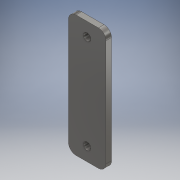
# Autodesk Inventor part: SIDE BEARING GUIDE
Saved by Autodesk Inventor 2018 (Build 220112000, 112)
## iProperties
Created: 2018-10-05
Part Number: SIDE BEARING GUIDE
Material: Acero
Document SubType Name: Modeling
Designer: Toshiba
Density: 7.85 g/cm^3
Appearance: Semipulido
Author: Toshiba
Autodesk Inventor part; units mm, degrees
ref_plane "YZ Plane" through (0, 0, 0) normal (1, 0, 0) x (0, 1, 0)
ref_plane "XZ Plane" through (0, 0, 0) normal (0, 1, 0) x (-1, 0, 0)
ref_plane "XY Plane" through (0, 0, 0) normal (0, 0, 1) x (1, 0, 0)
sketch "Boceto3" plane through (0, 0, 0) normal (0, 0, 1) x (1, 0, 0)
  line L0 (20, -3) -> (20, 3)
  line L1 (20, 3) -> (-20, 3)
  line L2 (-20, 3) -> (-20, -3)
  line L3 (-20, -3) -> (20, -3)
  line L4 (20, -3) -> (-20, 3) construction
  line L5 (20, 3) -> (-20, -3) construction
  point P0 (0, 0)
  dimension "d15" = 6
  dimension "d16" = 40
  constraints: 12 end point, 2 midpoint, 2 parallel, 1 perpendicular, 1 vertical
  measures "d15" distance of L0.start L0.end
  measures "d16" distance of L1.end L0.end
extrude "Extrusión3" add sketch "Boceto3" along normal mid plane 130
sketch "Boceto4" plane through (-20, 3, 65) normal (0, 1, 0) x (1, 0, 0)
  line L0 (35, 102.5) -> (35, 27.5)
  line L1 (35, 27.5) -> (5, 27.5)
  line L2 (5, 27.5) -> (5, 102.5)
  line L3 (5, 102.5) -> (35, 102.5)
  line L4 (35, 102.5) -> (5, 27.5) construction
  line L5 (35, 27.5) -> (5, 102.5) construction
  circle A0 centre (20, 14.5) radius 4
  circle A1 centre (20, 14.5) radius 13
  line L6 (14.6627, 65) -> (25.4742, 65)
  circle A2 centre (20, 115.5) radius 4
  circle A3 centre (20, 115.5) radius 13
  point P0 (20, 65)
  point P1 (20, 65)
  dimension "d19" = 75
  dimension "d20" = 8
  dimension "d21" = 26
  constraints: 14 end point, 4 centre point, 3 coincident, 2 midpoint, 2 parallel, 2 symmetric about line, 1 horizontal, 1 perpendicular, 1 point on line, 1 tangent, 1 vertical, 2 other
  measures "d19" distance of L0.start L0.end
  measures "d20" diameter of A0
  measures "d21" diameter of A1
extrude "Extrusión4" cut sketch "Boceto4" against normal through all contours A0 | A2
fillet "Empalme2" radius 8 4 edges at (20, 0, 65) (-20, 0, 65) (-20, 0, -65) (20, 0, -65)
